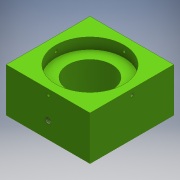
# Autodesk Inventor part: tubeLensHolder_v5
Saved by Autodesk Inventor 2016 (Build 200138000, 138)
## iProperties
Created: 2016-03-13
Part Number: tubeLensHolder_v5
Material: Generic
Document SubType Name: Modeling
Designer: sims01
Density: 1 g/cm^3
Appearance: Default
Author: sims01
Autodesk Inventor part; units mm, degrees
ref_plane "YZ Plane" through (0, 0, 0) normal (1, 0, 0) x (0, 1, 0)
ref_plane "XZ Plane" through (0, 0, 0) normal (0, 1, 0) x (-1, 0, 0)
ref_plane "XY Plane" through (0, 0, 0) normal (0, 0, 1) x (1, 0, 0)
sketch "Sketch1" plane through (0, 0, 0) normal (0, 0, 1) x (1, 0, 0)
  line L0 (-38.1, 38.1) -> (38.1, 38.1)
  line L1 (38.1, 38.1) -> (38.1, -38.1)
  line L2 (38.1, -38.1) -> (-38.1, -38.1)
  line L3 (-38.1, -38.1) -> (-38.1, 38.1)
  point P0 (0, 0)
  dimension "d0" = 76.2
  dimension "d1" = 76.2
  dimension "d2" = 38.1
  dimension "d3" = 38.1
  constraints: 8 end point, 2 parallel, 1 horizontal, 1 perpendicular
  measures "d0" distance of L0.end L1.end
  measures "d1" distance of L0.start L0.end
  measures "d2" distance from line of point (0, 0) L1
  measures "d3" distance from line of point (0, 0) L0
extrude "baseExtrusion" add sketch "Sketch1" along normal blind 40
sketch "Sketch2" plane through (0, 0, 40) normal (0, 0, 1) x (1, 0, 0)
  circle A0 centre (0, 0) radius 31
  dimension "d6" = 62
  constraints: 1 centre point, 1 coincident
  measures "d6" diameter of A0
extrude "tlExtrusion" cut sketch "Sketch2" against normal blind 10
sketch "Sketch3" plane through (0, 0, 0) normal (0, 0, -1) x (-1, 0, 0)
  circle A0 centre (0, 0) radius 20
  dimension "d9" = 40
  constraints: 1 centre point, 1 coincident
  measures "d9" diameter of A0
extrude "lightPathExtrusion" cut sketch "Sketch3" against normal through all
sketch "Sketch4" plane through (38.1, -38.1, 0) normal (1, 0, 0) x (0, 0, -1)
  line L0 (0, 76.2) -> (0, 0) projected
  line L1 (-40, 0) -> (-40, 76.2) projected
  point P0 (0, 38.1)
  point P1 (-35, 38.1)
  point P2 (0, 38.1)
  dimension "d12" = 5
  constraints: 1 horizontal alignment, 1 midpoint
  measures "d12" distance from line of point (-35, 38.1) L1
hole "tubeLensGrubScrew1" at (38.1, 0, 35) direction (-1, 0, 0) diameter 2.459 end through all thread size "M3x0.5" class "6H" standard "ISO Metric profile"
pattern_circular "tubeLensGrubScrew2" count 2 over 90 about axis through (0, 0, -10) along (0, 0, 1) of "tubeLensGrubScrew1"
sketch "Sketch5" plane through (0, 0, 0) normal (0, 0, -1) x (-1, 0, 0)
  point P0 (0, 0)
  point P1 (-30, -30)
  point P2 (-30, 30)
  point P3 (30, -30)
  point P4 (30, 30)
  dimension "d23" = 60
  dimension "d24" = 60
  dimension "d25" = 30
  dimension "d26" = 30
  constraints: 2 horizontal alignment, 2 vertical alignment
  measures "d23" distance of point (-30, 30) point (-30, -30)
  measures "d24" distance of point (30, 30) point (-30, 30)
  measures "d25" horizontal distance of point (0, 0) point (-30, 30)
  measures "d26" horizontal distance of point (0, 0) point (-30, 30)
hole "60mmCageSystem" at (30, -30, 0) at (30, 30, 0) at (-30, -30, 0) at (-30, 30, 0) direction (0, 0, 1) diameter 2.156 depth 10 tip angle 118 thread size "4-40 UNC" class "2B" standard "ANSI Unified Screw Threads"
sketch "Sketch6" plane through (-38.1, -38.1, 0) normal (0, -1, 0) x (1, 0, 0)
  line L0 (76.2, 0) -> (0, 0) projected
  point P0 (38.1, 0)
  point P1 (38.1, 15)
  point P2 (38.1, 0)
  dimension "d34" = 15
  constraints: 1 midpoint, 1 vertical alignment
  measures "d34" distance of point (38.1, 0) point (38.1, 15)
hole "m6MountingHole" at (0, -38.1, 15) direction (0, 1, 0) diameter 4.917 depth 15 tip angle 118 thread size "M6x1" class "6H" standard "ISO Metric profile"
equation "\"d2\" = 0.5 * d1"
equation "\"d3\" = 0.5 * d0"
equation "\"d25\" = 0.5 * d23"
equation "\"d26\" = 0.5 * d24"
body "Solid1"
